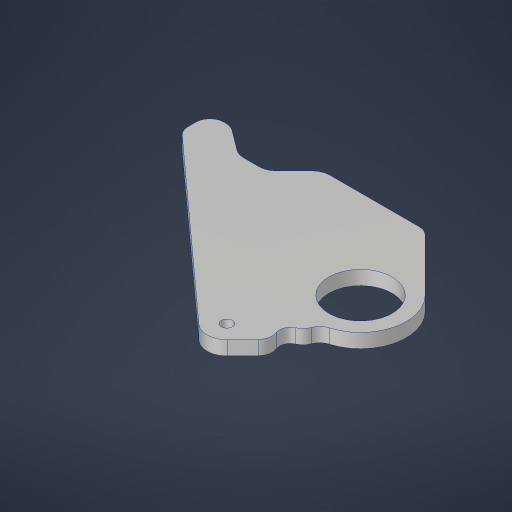
# Autodesk Inventor part: CL5-003
Saved by Autodesk Inventor 2023.4 (Build 274418000, 418)
## iProperties
Created: 2025-02-03
Part Number: CL5-003
Material: Aluminum 6061
Document SubType Name: Modeling
Designer: brand
Density: 2.7 g/cm^3
Appearance: Aluminum - Flat
Author: brand
Autodesk Inventor part; units mm, degrees
ref_plane "YZ Plane" through (0, 0, 0) normal (1, 0, 0) x (0, 1, 0)
ref_plane "XZ Plane" through (0, 0, 0) normal (0, 1, 0) x (-1, 0, 0)
ref_plane "XY Plane" through (0, 0, 0) normal (0, 0, 1) x (1, 0, 0)
sketch "Sketch1" plane through (0, 0, 0) normal (0, 1, 0) x (-1, 0, 0)
  circle A0 centre (76.2, -63.1164) radius 16.7005 construction
  line L0 (69.85, -27.2929) -> (82.55, -27.2929)
  line L1 (82.55, -27.2929) -> (95.25, -36.8179)
  line L2 (95.25, -36.8179) -> (104.775, -36.8179)
  line L3 (104.775, -36.8179) -> (104.775, -24.1179)
  line L4 (104.775, -24.1179) -> (25.0156, 47.8833)
  line L5 (69.85, -27.2929) -> (57.15, -39.9929)
  line L6 (57.15, -39.9929) -> (10.8071, -39.9929)
  circle A1 centre (0, 0) radius 14.2875
  circle A2 centre (0, 0) radius 20.6375 construction
  line L7 (10.8071, -39.9929) -> (-14.5929, -14.5929)
  circle A3 centre (0, 31.75) radius 4.7625 construction
  circle A4 centre (19.05, 41.275) radius 2.5527 construction
  circle A5 centre (19.05, 41.275) radius 8.9027 construction
  line L8 (12.6625, 47.4764) -> (1.7098, 36.195)
  arc A6 (-1.27, 27.16) -> (1.7098, 36.195) centre (0, 31.75) ccw
  arc A7 (1.27, 20.5984) -> (-14.5929, -14.5929) centre (0, 0) ccw
  arc A8 (25.0156, 47.8833) -> (12.6625, 47.4764) centre (19.05, 41.275) ccw
  line L9 (-1.27, 27.16) -> (1.27, 20.5984)
  point P0 (76.2, -27.2929)
  dimension "d0" = 33.401
  dimension "d1" = 28.575
  dimension "d2" = 6.35
  dimension "d3" = 9.525
  dimension "d4" = 31.75
  dimension "d5" = 5.1054
  dimension "d6" = 6.35
  dimension "d7" = 19.05
  dimension "d8" = 9.525
  dimension "d9" = 25.4
  dimension "d10" = 25.4
  dimension "d11" = 12.7
  dimension "d12" = 12.7
  dimension "d13" = 12.7
  dimension "d15" = 76.2
  dimension "d16" = 76.2
  dimension "d17" = 12.7
  dimension "d18" = 3.175
  dimension "d19" = 9.525
  dimension "d20" = 12.7
  dimension "d34" = 4.445
  dimension "d35" = 1.27
  dimension "d36" = 1.27
  constraints: 20 end point, 10 point on circle, 8 centre point, 4 coincident, 2 horizontal, 2 tangent, 1 concentric, 1 midpoint, 1 parallel, 1 vertical, 1 vertical alignment, 4 other
  measures "d0" diameter of A0
  measures "d1" diameter of A1
  measures "d3" diameter of A3
  measures "d4" distance of A3.centre point (0, 0)
  measures "d5" diameter of A4
  measures "d6" radial gap between concentric circles of A4 A5
  measures "d7" horizontal distance of A4.centre A3.centre
  measures "d8" vertical distance of A3.centre A4.centre
  measures "d9" horizontal distance of L7.end L6.end
  measures "d10" horizontal distance of L7.end L6.end
  measures "d11" horizontal distance of L0.start L5.end
  measures "d12" horizontal distance of L0.start L5.end
  measures "d13" distance of L0.start L0.end
  measures "d15" horizontal distance of point (0, 0) point (76.2, -27.293)
  measures "d16" horizontal distance of point (0, 0) A0.centre
  measures "d17" horizontal distance of L0.end L1.end
  measures "d18" distance between parallel lines of L6 L2
  measures "d19" distance of L1.end L2.end
  measures "d20" distance of L2.end L3.end
  measures "d34" vertical distance of A3.centre L8.end
  measures "d35" horizontal distance of A3.centre L9.start
  measures "d36" horizontal distance of point (0, 0) L9.end
extrude "Extrusion1" add sketch "Sketch1" against normal blind 6.35
fillet "Fillet1" radius 6.35 6 edges at (-1.7098, -3.175, 36.195) (-10.8071, -3.175, -39.9929) (-104.775, -3.175, -24.1179) (-104.775, -3.175, -36.8179) (1.27, -3.175, 27.16) (-1.27, -3.175, 20.5984)
fillet "Fillet2" radius 7.62 4 edges at (-69.85, -3.175, -27.2929) (-82.55, -3.175, -27.2929) (-57.15, -3.175, -39.9929) (-95.25, -3.175, -36.8179)
hole "Hole1" at (-19.05, 0, 41.275) direction (0, -1, 0) diameter 5.1054 end through all clearance for "Flat Head Machine Screw (82)" size "#10" standard "Ansi Unified Screw Threads"
equation "\"d17\" = d12"
body "Solid1"
